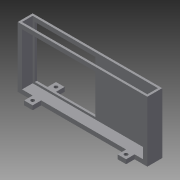
# Autodesk Inventor part: PhoneCase
Saved by Autodesk Inventor 2015 (Build 190159000, 159)
## iProperties
Created: 2015-04-29
Part Number: PhoneCase
Material: Generic
Document SubType Name: Modeling
Designer: 166348
Density: 1 g/cm^3
Appearance: Default
Author: 166348
Autodesk Inventor part; units mm, degrees
ref_plane "YZ Plane" through (0, 0, 0) normal (1, 0, 0) x (0, 1, 0)
ref_plane "XZ Plane" through (0, 0, 0) normal (0, 1, 0) x (-1, 0, 0)
ref_plane "XY Plane" through (0, 0, 0) normal (0, 0, 1) x (1, 0, 0)
sketch "Sketch1" plane through (0, 0, 0) normal (0, 0, 1) x (1, 0, 0)
  line L0 (0, 0) -> (0, 67.31)
  line L1 (0, 67.31) -> (149.86, 67.31)
  line L2 (149.86, 67.31) -> (149.86, 0)
  line L3 (149.86, 0) -> (0, 0)
  line L4 (-2.54, 69.85) -> (-2.54, -2.54)
  line L5 (-2.54, -2.54) -> (152.4, -2.54)
  line L6 (152.4, -2.54) -> (152.4, 69.85)
  line L7 (152.4, 69.85) -> (-2.54, 69.85)
  dimension "d0" = 67.31
  dimension "d1" = 149.86
  dimension "d5" = 72.39
  dimension "d6" = 154.94
  dimension "d7" = 72.39
  constraints: 16 end point, 4 perpendicular, 3 vertical
  measures "d0" distance of L0.start L0.end
  measures "d1" distance of L0.end L1.end
  measures "d5" distance of L4.start L4.end
  measures "d6" distance of L4.end L5.end
  measures "d7" distance of L5.end L6.end
extrude "Extrusion1" add sketch "Sketch1" along normal blind 17.78
sketch "Sketch2" plane through (0, 0, 0) normal (1, 0, 0) x (0, 0, -1)
  line L0 (0, 0) -> (-2.54, 0)
  line L1 (0, 0) -> (-17.78, 0) projected
  line L2 (-2.54, 0) -> (-2.54, 67.31)
  line L3 (0, 67.31) -> (-17.78, 67.31) projected
  line L4 (-2.54, 67.31) -> (0, 67.31)
  line L5 (0, 67.31) -> (0, 0)
  line L6 (0, 67.31) -> (0, 0) projected
  dimension "d10" = 2.54
  constraints: 8 end point, 2 point on line, 1 collinear, 1 horizontal, 1 perpendicular
  measures "d10" distance of L0.start L0.end
extrude "Extrusion2" add sketch "Sketch2" along normal blind 2.54
sketch "Sketch3" plane through (0, 0, 17.78) normal (0, 1, 0) x (1, 0, 0)
  line L0 (0, 15.24) -> (0, 0) projected
  line L1 (0, 2.54) -> (149.86, 2.54)
  line L2 (149.86, 2.54) -> (149.86, 0)
  line L3 (149.86, 0) -> (0, 0)
  line L4 (0, 0) -> (149.86, 0) projected
  point P0 (0, 17.78)
  constraints: 6 end point, 1 collinear, 1 horizontal, 1 point on line, 1 vertical
extrude "Extrusion3" add sketch "Sketch3" along normal blind 2.54
sketch "Sketch4" plane through (-2.54, 69.85, 0) normal (0, 1, 0) x (1, 0, 0)
  line L0 (2.54, -15.24) -> (2.54, -2.54)
  line L1 (2.54, -2.54) -> (2.54, -15.24) projected
  line L2 (2.54, -2.54) -> (152.4, -2.54)
  line L3 (152.4, 0) -> (152.4, -15.24) projected
  line L4 (152.4, -15.24) -> (2.54, -15.24)
  point P0 (2.54, 0)
  constraints: 6 end point, 2 perpendicular, 1 collinear, 1 point on line
extrude "Extrusion4" cut sketch "Sketch4" against normal blind 2.54
sketch "Sketch5" plane through (0, 67.31, 17.78) normal (0, -1, 0) x (1, 0, 0)
  line L0 (149.86, 0) -> (149.86, -2.54)
  line L1 (149.86, -2.54) -> (0, -2.54)
  line L2 (0, -2.54) -> (0, 0)
  line L3 (0, 0) -> (149.86, 0)
  point P0 (0, -17.78)
  constraints: 8 end point, 3 perpendicular, 1 vertical
extrude "Extrusion5" add sketch "Sketch5" along normal blind 2.54
sketch "Sketch6" plane through (0, 0, 2.54) normal (1, 0, 0) x (0, 0, -1)
  line L0 (-12.7, 2.54) -> (-15.24, 2.54)
  line L1 (-15.24, 2.54) -> (-15.24, 64.77)
  line L2 (-15.24, -2.54) -> (-15.24, 69.85) projected
  line L3 (-15.24, 64.77) -> (-12.7, 64.77)
  line L4 (-12.7, 64.77) -> (-12.7, 2.54)
  point P0 (2.54, 0)
  dimension "d19" = 62.23
  constraints: 8 end point, 1 horizontal, 1 parallel, 1 perpendicular, 1 point on line
  measures "d19" distance of L0.end L1.end
extrude "Extrusion6" add sketch "Sketch6" along normal blind 2.54
sketch "Sketch7" plane through (0, 2.54, 17.78) normal (0, 1, 0) x (1, 0, 0)
  line L0 (149.86, 2.54) -> (149.86, 0)
  line L1 (149.86, 0) -> (147.32, 0)
  line L2 (149.86, 0) -> (2.54, 0) projected
  line L3 (147.32, 0) -> (147.32, 2.54)
  line L4 (147.32, 2.54) -> (149.86, 2.54)
  point P0 (0, 17.78)
  dimension "d22" = 2.54
  constraints: 8 end point, 2 perpendicular, 1 point on line, 1 vertical
  measures "d22" distance of L0.end L1.end
extrude "Extrusion7" add sketch "Sketch7" along normal blind 62.23
sketch "Sketch8" plane through (149.86, 0, 0) normal (-1, 0, 0) x (0, 0, 1)
  line L0 (0, 0) -> (2.54, 0)
  line L1 (2.54, 0) -> (2.54, 2.54)
  line L2 (2.54, 69.85) -> (2.54, 0) projected
  line L3 (2.54, 2.54) -> (0, 2.54)
  line L4 (0, 0) -> (0, 67.31) projected
  dimension "d25" = 2.54
  constraints: 6 end point, 2 point on line, 1 horizontal, 1 perpendicular
  measures "d25" distance of L0.end L1.end
extrude "Extrusion8" add sketch "Sketch8" along normal blind 149.86
sketch "Sketch9" plane through (149.86, 67.31, 2.54) normal (-1, 0, 0) x (0, 0, 1)
  line L0 (-2.54, 0) -> (0, 0)
  line L1 (0, 0) -> (0, -2.54)
  line L2 (0, 0) -> (0, -64.77) projected
  line L3 (0, -2.54) -> (-2.54, -2.54)
  line L4 (-2.54, -64.77) -> (-2.54, 0) projected
  point P0 (-2.54, -67.31)
  point P1 (0, -67.31)
  dimension "d28" = 2.54
  dimension "d29" = 2.54
  constraints: 6 end point, 2 point on line, 1 horizontal, 1 perpendicular
  measures "d28" distance of L0.start L0.end
  measures "d29" distance of L0.end L1.end
extrude "Extrusion9" add sketch "Sketch9" along normal blind 149.86
sketch "Sketch10" plane through (149.86, 0, 15.24) normal (-1, 0, 0) x (0, 0, 1)
  line L0 (-15.24, 2.54) -> (-12.7, 2.54)
  line L1 (-12.7, 2.54) -> (-12.7, 64.77)
  line L2 (-12.7, 64.77) -> (-15.24, 64.77)
  line L3 (-15.24, -2.54) -> (-15.24, 69.85) projected
  point P0 (-15.24, 0)
  constraints: 6 end point, 2 perpendicular, 1 horizontal, 1 point on line
extrude "Extrusion10" add sketch "Sketch10" along normal blind 74.93
sketch "Sketch11" plane through (0, 0, 17.78) normal (0, 0, 1) x (1, 0, 0)
  line L0 (147.32, 2.54) -> (2.54, 2.54) projected
  line L1 (15.24, 2.54) -> (15.24, -2.54)
  line L2 (-2.54, -2.54) -> (152.4, -2.54) projected
  line L3 (15.24, -2.54) -> (25.4, -2.54)
  line L4 (25.4, -2.54) -> (25.4, 2.54)
  point P0 (0, 0)
  dimension "d34" = 10.16
  constraints: 6 end point, 4 point on line, 1 perpendicular, 1 vertical
  measures "d34" distance of L1.end L3.end
extrude "Extrusion11" add sketch "Sketch11" along normal blind 10.16
sketch "Sketch12" plane through (0, 2.54, 17.78) normal (0, 1, 0) x (1, 0, 0)
  line L0 (15.24, 0) -> (15.24, -5.08)
  line L1 (15.24, 0) -> (15.24, -10.16) projected
  line L2 (15.24, -5.08) -> (20.32, -5.08)
  circle A0 centre (20.32, -5.08) radius 2.159
  point P0 (0, 17.78)
  dimension "d37" = 5.08
  dimension "d38" = 5.08
  dimension "d39" = 4.318
  constraints: 4 end point, 1 centre point, 1 coincident, 1 midpoint, 1 perpendicular
  measures "d37" distance of L0.start L0.end
  measures "d38" distance of L0.end L2.end
  measures "d39" diameter of A0
extrude "Extrusion12" cut sketch "Sketch12" against normal blind 10.16
sketch "Sketch13" plane through (0, 0, 17.78) normal (0, 0, 1) x (1, 0, 0)
  line L0 (149.86, 0) -> (137.16, 0)
  line L1 (0, 0) -> (149.86, 0) projected
  line L2 (137.16, 0) -> (137.16, 2.54)
  line L3 (147.32, 2.54) -> (2.54, 2.54) projected
  line L4 (137.16, 2.54) -> (127, 2.54)
  line L5 (127, 2.54) -> (127, -2.54)
  line L6 (25.4, -2.54) -> (152.4, -2.54) projected
  line L7 (137.16, -2.54) -> (137.16, 0)
  dimension "d42" = 12.7
  dimension "d43" = 10.16
  constraints: 10 end point, 6 point on line, 3 perpendicular
  measures "d42" distance of L0.start L0.end
  measures "d43" distance of L2.end L4.end
extrude "Extrusion13" add sketch "Sketch13" along normal blind 10.16
sketch "Sketch14" plane through (0, 2.54, 17.78) normal (0, 1, 0) x (1, 0, 0)
  line L0 (127, 0) -> (127, -5.08)
  line L1 (127, 0) -> (127, -10.16) projected
  line L2 (127, -5.08) -> (132.08, -5.08)
  circle A0 centre (132.08, -5.08) radius 2.159
  point P0 (0, 17.78)
  dimension "d46" = 5.08
  dimension "d47" = 5.08
  dimension "d48" = 4.318
  constraints: 4 end point, 1 centre point, 1 coincident, 1 midpoint, 1 perpendicular
  measures "d46" distance of L0.start L0.end
  measures "d47" distance of L0.end L2.end
  measures "d48" diameter of A0
extrude "Extrusion14" cut sketch "Sketch14" against normal blind 10.16
sketch "Sketch15" plane through (0, 0, 0) normal (0, 0, -1) x (-1, 0, 0)
  line L0 (0, 0) -> (-149.86, 0) projected
  line L1 (-15.24, 0) -> (-15.24, 2.54)
  line L2 (-74.93, 2.54) -> (-2.54, 2.54) projected
  line L3 (-15.24, 2.54) -> (-25.4, 2.54)
  line L4 (-25.4, 2.54) -> (-25.4, -2.54)
  line L5 (-15.24, -2.54) -> (-25.4, -2.54) projected
  line L6 (-25.4, -2.54) -> (-15.24, -2.54)
  line L7 (-15.24, -2.54) -> (-15.24, 2.54)
  dimension "d51" = 10.16
  constraints: 10 end point, 4 point on line, 2 perpendicular, 1 collinear, 1 vertical
  measures "d51" distance of L1.end L3.end
extrude "Extrusion15" add sketch "Sketch15" along normal blind 10.16
sketch "Sketch16" plane through (2.54, 2.54, 2.54) normal (0, 1, 0) x (1, 0, 0)
  line L0 (12.7, 2.54) -> (12.7, 7.62)
  line L1 (12.7, 2.54) -> (12.7, 12.7) projected
  line L2 (12.7, 7.62) -> (17.78, 7.62)
  circle A0 centre (17.78, 7.62) radius 2.159
  point P0 (-2.54, 2.54)
  dimension "d54" = 5.08
  dimension "d55" = 5.08
  dimension "d56" = 4.318
  constraints: 4 end point, 1 centre point, 1 coincident, 1 midpoint, 1 perpendicular
  measures "d54" distance of L0.start L0.end
  measures "d55" distance of L0.end L2.end
  measures "d56" diameter of A0
extrude "Extrusion16" cut sketch "Sketch16" against normal blind 10.16
sketch "Sketch17" plane through (0, 0, 0) normal (0, 0, -1) x (-1, 0, 0)
  line L0 (-149.86, 69.85) -> (-149.86, 0) projected
  line L1 (-149.86, 2.54) -> (-137.16, 2.54)
  line L2 (-137.16, 2.54) -> (-147.32, 2.54) projected
  line L3 (-137.16, 2.54) -> (-137.16, -2.54)
  line L4 (0, 0) -> (-149.86, 0) projected
  line L5 (-137.16, -2.54) -> (-127, -2.54)
  line L6 (-127, -2.54) -> (-137.16, -2.54) projected
  line L7 (-127, -2.54) -> (-127, 2.54)
  line L8 (-127, 2.54) -> (-137.16, 2.54)
  line L9 (-137.16, 2.54) -> (-127, 2.54) projected
  dimension "d59" = 12.7
  dimension "d60" = 10.16
  constraints: 10 end point, 3 collinear, 2 perpendicular, 1 point on line
  measures "d59" distance of L1.start L1.end
  measures "d60" distance of L3.end L5.end
extrude "Extrusion17" add sketch "Sketch17" along normal blind 10.16 contours L4 L7 L5 L3 | L3 L8 L7 L4
sketch "Sketch18" plane through (127, 2.54, 0) normal (0, 1, 0) x (1, 0, 0)
  line L0 (0, 0) -> (0, 5.08)
  line L1 (0, 0) -> (0, 10.16) projected
  line L2 (0, 5.08) -> (5.08, 5.08)
  circle A0 centre (5.08, 5.08) radius 2.159
  point P0 (-127, 0)
  dimension "d63" = 5.08
  dimension "d64" = 5.08
  dimension "d65" = 4.318
  constraints: 4 end point, 1 centre point, 1 coincident, 1 midpoint, 1 perpendicular
  measures "d63" distance of L0.start L0.end
  measures "d64" distance of L0.end L2.end
  measures "d65" diameter of A0
extrude "Extrusion18" cut sketch "Sketch18" against normal blind 10.16
body "Solid1"
